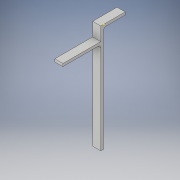
# Autodesk Inventor part: RightTopPlateConnector
Saved by Autodesk Inventor 2017 (Build 210142000, 142)
## iProperties
Created: 2017-12-13
Part Number: RightTopPlateConnector
Material: Generic
Document SubType Name: Modeling
Designer: User
Density: 1 g/cm^3
Appearance: Default
Author: User
Autodesk Inventor part; units mm, degrees
ref_plane "YZ Plane" through (0, 0, 0) normal (1, 0, 0) x (0, 1, 0)
ref_plane "XZ Plane" through (0, 0, 0) normal (0, 1, 0) x (-1, 0, 0)
ref_plane "XY Plane" through (0, 0, 0) normal (0, 0, 1) x (1, 0, 0)
sketch "Sketch3" plane through (0, 0, 0) normal (0, 0, 1) x (1, 0, 0)
  line L0 (0, 0) -> (19.05, 0)
  line L1 (19.05, 0) -> (19.05, -254)
  line L2 (19.05, -254) -> (0, -254)
  line L3 (0, -254) -> (0, 0)
  dimension "d0" = 19.05
  dimension "d1" = 254
  constraints: 8 end point, 2 parallel, 1 horizontal, 1 perpendicular
  measures "d0" distance of L1.end L2.end
  measures "d1" distance of L0.end L1.end
extrude "Extrusion1" add sketch "Sketch3" along normal blind 6.35
sketch "Sketch4" plane through (19.05, -254, 0) normal (1, 0, 0) x (0, 0, -1)
  point P0 (0, 254)
sketch "Sketch5" plane through (0, 0, 6.35) normal (0, 0, 1) x (1, 0, 0)
  line L0 (19.05, 0) -> (0, 0) projected
  line L1 (0, 0) -> (0, -31.75)
  line L2 (0, 0) -> (0, -254) projected
  line L3 (19.05, -254) -> (19.05, 0) projected
  line L4 (0, -31.75) -> (19.05, -31.75)
  line L5 (19.05, -31.75) -> (19.05, -38.1)
  line L6 (19.05, -38.1) -> (0, -38.1)
  line L7 (0, -38.1) -> (0, -31.75)
  dimension "d4" = 31.75
  dimension "d5" = 6.35
  constraints: 10 end point, 2 parallel, 2 point on line, 1 horizontal, 1 perpendicular
  measures "d4" distance of L0.end L1.end
  measures "d5" distance of L4.end L5.end
extrude "Extrusion2" add sketch "Sketch5" along normal blind 88.9 contours L3 L6 L2 L4
sketch "Sketch6" plane through (0, 0, 0) normal (0, 0, -1) x (-1, 0, 0)
  line L0 (-19.05, -31.75) -> (-19.05, 0) projected
  line L1 (0, 0) -> (-19.05, 0)
  line L2 (-19.05, 0) -> (-19.05, -6.35)
  line L3 (-19.05, -6.35) -> (0, -6.35)
  line L4 (0, -6.35) -> (0, 0)
  dimension "d8" = 6.35
  constraints: 8 end point, 2 parallel, 1 horizontal, 1 perpendicular, 1 point on line
  measures "d8" distance of L2.end L1.end
extrude "Extrusion3" add sketch "Sketch6" along normal blind 50.8
fillet "Fillet2" radius 6.35 2 edges at (9.525, -38.1, 6.35) (9.525, -6.35, 0)
body "Solid1"
